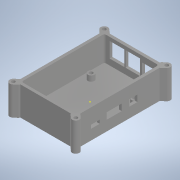
# Autodesk Inventor part: Case Rev D
Saved by Autodesk Inventor 2021 (Build 250183000, 183)
## iProperties
Created: 2021-07-24
Part Number: Case Rev D
Material: ABS Plastic
Document SubType Name: Modeling
Designer: cmzgt
Density: 0.1 g/cm^3
Appearance: Smooth - White
Author: cmzgt
Autodesk Inventor part; units mm, degrees
ref_plane "YZ Plane" through (0, 0, 0) normal (1, 0, 0) x (0, 1, 0)
ref_plane "XZ Plane" through (0, 0, 0) normal (0, 1, 0) x (-1, 0, 0)
ref_plane "XY Plane" through (0, 0, 0) normal (0, 0, 1) x (1, 0, 0)
sketch "Sketch1" plane through (0, 0, 0) normal (0, 1, 0) x (-1, 0, 0)
  line L0 (-33.8, -50.05) -> (33.8, -50.05)
  line L1 (33.8, -50.05) -> (33.8, 50.05)
  line L2 (33.8, 50.05) -> (-33.8, 50.05)
  line L3 (-33.8, 50.05) -> (-33.8, -50.05)
  line L4 (-33.8, -50.05) -> (33.8, 50.05) construction
  line L5 (33.8, -50.05) -> (-33.8, 50.05) construction
  point P0 (0, 0)
  dimension "d0" = 67.6
  dimension "d1" = 100.1
  constraints: 12 end point, 2 midpoint, 2 parallel, 1 horizontal, 1 perpendicular
  measures "d0" distance of L2.end L1.end
  measures "d1" distance of L0.end L1.end
extrude "Extrusion1" add sketch "Sketch1" along normal blind 4.445
sketch "Sketch2" plane through (0, 4.445, 0) normal (0, 1, 0) x (1, 0, 0)
  line L0 (30.6, 46.85) -> (-30.6, 46.85)
  line L1 (-30.6, 46.85) -> (-30.6, -46.85)
  line L2 (-30.6, -46.85) -> (30.6, -46.85)
  line L3 (30.6, -46.85) -> (30.6, 46.85)
  line L4 (30.6, 46.85) -> (-30.6, -46.85) construction
  line L5 (-30.6, 46.85) -> (30.6, -46.85) construction
  line L6 (-33.8, 50.05) -> (-33.8, -50.05) projected
  line L7 (-33.8, -50.05) -> (33.8, -50.05) projected
  line L8 (33.8, 50.05) -> (-33.8, 50.05) projected
  line L9 (33.8, -50.05) -> (33.8, 50.05) projected
  line L10 (27.4, -43.65) -> (33.8, -50.05) construction
  line L11 (24.9431, -46.85) -> (30.9716, -52.8784)
  line L12 (36.6284, -47.2216) -> (30.6, -41.1931)
  arc A0 (30.9716, -52.8784) -> (36.6284, -47.2216) centre (33.8, -50.05) ccw
  circle A1 centre (33.8, -50.05) radius 1.375
  point P0 (0, 0)
  dimension "d4" = 3.2
  dimension "d5" = 3.2
  dimension "d22" = 8
  dimension "d23" = 2.75
  constraints: 20 end point, 4 parallel, 3 midpoint, 2 centre point, 2 point on circle, 2 point on line, 2 tangent, 1 coincident, 1 horizontal, 1 perpendicular
  measures "d4" distance between parallel lines of L6 L1
  measures "d5" distance between parallel lines of L7 L2
  measures "d22" diameter of A0
  measures "d23" diameter of A1
extrude "Extrusion2" add sketch "Sketch2" along normal blind 28 contours L0 L1 L2 L11 L7 L6 L8 L9 L12 L3 | L12 L9 A1 L7 L11 L2 L3 | L9 L7 A1 picked at (32.9402, -49.7491)
sketch "Sketch4" plane through (0, 0, 0) normal (0, -1, 0) x (1, 0, 0)
  line L0 (32.2906, 48.7379) -> (35.3094, 51.3621) construction
  line L1 (33.8, 50.05) -> (33.8, -50.05) projected
  line L2 (33.8, 44.7499) -> (37.9337, 48.3433)
  line L3 (32.6852, 54.381) -> (29.6663, 51.7567)
  arc A0 (29.6663, 51.7567) -> (28.5119, 50.05) centre (32.2906, 48.7379) ccw
  arc A1 (37.9337, 48.3433) -> (32.6852, 54.381) centre (35.3094, 51.3621) ccw
  line L4 (-33.8, 50.05) -> (33.8, 50.05) projected
  line L5 (28.5119, 50.05) -> (33.8, 50.05)
  line L6 (33.8, 50.05) -> (33.8, 44.7499)
  circle A2 centre (35.3094, 51.3621) radius 1.985
  line L7 (0, 50.05) -> (0, -50.05) construction
  line L8 (33.8, -50.05) -> (-33.8, -50.05) construction
  line L9 (33.8, 0) -> (-33.3, 0) construction
  line L10 (33.8, -50.05) -> (33.8, 50.05)
  line L11 (33.8, -44.7499) -> (37.9337, -48.3433)
  line L12 (32.6852, -54.381) -> (29.6663, -51.7567)
  arc A3 (28.5119, -50.05) -> (29.6663, -51.7567) centre (32.2906, -48.7379) ccw
  arc A4 (32.6852, -54.381) -> (37.9337, -48.3433) centre (35.3094, -51.3621) ccw
  line L13 (-33.8, -50.05) -> (33.8, -50.05)
  circle A5 centre (35.3094, -51.3621) radius 1.985
  line L14 (-33.8, 50.05) -> (-33.8, -50.05)
  line L15 (-33.8, 44.7499) -> (-37.9337, 48.3433)
  line L16 (-32.6852, 54.381) -> (-29.6663, 51.7567)
  arc A6 (-28.5119, 50.05) -> (-29.6663, 51.7567) centre (-32.2906, 48.7379) ccw
  arc A7 (-32.6852, 54.381) -> (-37.9337, 48.3433) centre (-35.3094, 51.3621) ccw
  line L17 (-28.5119, 50.05) -> (-33.8, 50.05)
  circle A8 centre (-35.3094, 51.3621) radius 1.985
  arc A9 (-37.9337, -48.3433) -> (-32.6852, -54.381) centre (-35.3094, -51.3621) ccw
  line L18 (-33.8, -44.7499) -> (-37.9337, -48.3433)
  line L19 (-32.6852, -54.381) -> (-29.6663, -51.7567)
  arc A10 (-29.6663, -51.7567) -> (-28.5119, -50.05) centre (-32.2906, -48.7379) ccw
  circle A11 centre (-35.3094, -51.3621) radius 1.985
  line L20 (-28.5119, -50.05) -> (-33.8, -50.05)
  line L21 (-33.8, -50.05) -> (-33.8, 50.05)
  point P0 (0, 0)
  point P1 (-28.5119, -50.05)
  point P2 (-33.8, -44.7499)
  point P3 (-28.5119, 50.05)
  point P4 (33.8, -44.7499)
  dimension "d24" = 2
  dimension "d25" = 8
  dimension "d26" = 131
  dimension "d27" = 3.97
  constraints: 40 end point, 30 symmetric about line, 16 point on circle, 12 centre point, 6 point on line, 4 coincident, 4 midpoint, 4 tangent, 1 collinear, 1 horizontal, 1 parallel, 9 other
  measures "d24" distance of L1.start L0.end
  measures "d25" diameter of A1
  measures "d26" angle of L1 L2
  measures "d27" diameter of A2
extrude "Extrusion4" add sketch "Sketch4" against normal up to surface (32.445 mm away) contours L4 A0 L3 A1 L2 L1 | L11 A4 L12 A3 L13 L1 | L4 L14 L15 A7 L16 A6 | A10 L19 A9 L18 L14 L13
fillet "Fillet2" radius 2 4 edges at (30.6, 18.445, -46.85) (-30.6, 18.445, -46.85) (-30.6, 18.445, 46.85) (30.6, 18.445, 46.85)
sketch "Sketch14" plane through (0, 4.445, 0) normal (0, 1, 0) x (1, 0, 0)
  circle A0 centre (27.1, -34.85) radius 3.7
  circle A1 centre (27.1, -34.85) radius 1.985
  line L0 (28.6, -46.85) -> (-28.6, -46.85) projected
  line L1 (30.6, 44.85) -> (30.6, -44.85) projected
  line L2 (-28.6, -46.85) -> (28.6, -46.85) construction
  line L3 (0, -46.85) -> (0, 50.05) construction
  line L4 (28.5119, 50.05) -> (-28.5119, 50.05) construction
  circle A2 centre (27.1, 23.15) radius 3.7
  circle A3 centre (27.1, 23.15) radius 1.985
  line L5 (-30.6, 44.85) -> (-30.6, -44.85) construction
  line L6 (-30.6, 0) -> (30.6, 0) construction
  line L7 (30.6, -44.85) -> (30.6, 44.85) construction
  circle A4 centre (-21.9, -34.85) radius 3.7
  circle A5 centre (-21.9, -34.85) radius 1.985
  circle A6 centre (-21.9, 23.15) radius 1.985
  circle A7 centre (-21.9, 23.15) radius 3.7
  point P0 (0, 0)
  dimension "d114" = 7.4
  dimension "d115" = 3.97
  dimension "d116" = 12
  dimension "d117" = 3.5
  dimension "d120" = 58
  dimension "d127" = 49
  constraints: 8 centre point, 4 coincident, 4 end point, 4 midpoint, 1 horizontal, 1 vertical, 12 other
  measures "d114" diameter of A0
  measures "d115" diameter of A1
  measures "d116" distance from line of L0 A0.centre
  measures "d117" distance from line of L1 A0.centre
  measures "d120" distance of A0.centre A2.centre
  measures "d127" distance of A0.centre A4.centre
sketch "Sketch15" plane through (0, 4.445, 0) normal (0, 1, 0) x (1, 0, 0)
  point P0 (0, 0)
extrude "Extrusion10" add sketch "Sketch14" along normal blind 6
sketch "Sketch16" plane through (33.8, 0, 44.7499) normal (1, 0, 0) x (0, 0, -1)
  line L0 (12.9515, 13.2621) -> (12.9515, 13.455) projected
  line L1 (20.9323, 13.455) -> (20.9323, 13.2621) projected
  line L2 (13.9419, 14.5004) -> (19.9419, 14.5004) projected
  line L3 (88.3241, 11.975) -> (9.3999, 11.975) projected
  line L4 (21.9323, 11.475) -> (11.9515, 11.475)
  line L5 (11.9515, 11.475) -> (11.9515, 15.5004)
  line L6 (11.9515, 15.5004) -> (21.9323, 15.5004)
  line L7 (21.9323, 15.5004) -> (21.9323, 11.475)
  line L8 (30.8419, 17.055) -> (30.8419, 14.5766) projected
  line L9 (45.8419, 14.5766) -> (45.8419, 17.055) projected
  line L10 (45.0419, 17.855) -> (31.6419, 17.855) projected
  line L11 (46.8419, 11.475) -> (29.8419, 11.475)
  line L12 (29.8419, 11.475) -> (29.8419, 18.855)
  line L13 (29.8419, 18.855) -> (46.8419, 18.855)
  line L14 (46.8419, 18.855) -> (46.8419, 11.475)
  line L15 (56.4419, 17.775) -> (56.4419, 11.775) projected
  line L16 (63.4419, 11.775) -> (63.4419, 17.775) projected
  line L17 (63.4419, 17.775) -> (59.9419, 17.775) projected
  line L18 (59.9419, 17.775) -> (56.4419, 17.775) projected
  line L19 (64.4419, 11.475) -> (55.4419, 11.475)
  line L20 (55.4419, 11.475) -> (55.4419, 18.775)
  line L21 (55.4419, 18.775) -> (64.4419, 18.775)
  line L22 (64.4419, 18.775) -> (64.4419, 11.475)
  point P0 (44.7499, 0)
  dimension "d134" = 1
  dimension "d135" = 0.5
  dimension "d136" = 1
  dimension "d137" = 1
  dimension "d138" = 1
  dimension "d139" = 0.5
  dimension "d140" = 1
  dimension "d141" = 1
  dimension "d142" = 0.5
  dimension "d143" = 1
  dimension "d144" = 1
  dimension "d145" = 1
  constraints: 24 end point, 6 parallel, 3 horizontal, 3 perpendicular
  measures "d134" distance between parallel lines of L2 L6
  measures "d135" distance between parallel lines of L3 L4
  measures "d136" distance between parallel lines of L1 L7
  measures "d137" distance between parallel lines of L5 L0
  measures "d138" distance between parallel lines of L13 L10
  measures "d139" distance between parallel lines of L3 L11
  measures "d140" distance between parallel lines of L9 L14
  measures "d141" distance from line of L8.end L12
  measures "d142" distance between parallel lines of L3 L19
  measures "d143" distance between parallel lines of L16 L22
  measures "d144" distance between parallel lines of L15 L20
  measures "d145" distance between parallel lines of L18 L21
extrude "Extrusion11" cut sketch "Sketch16" against normal up to surface (3.2 mm away)
sketch "Sketch17" plane through (28.5119, 0, -50.05) normal (0, 0, -1) x (-1, 0, 0)
  line L0 (16.1912, 11.975) -> (16.1912, 25.475) projected
  line L1 (0.3112, 11.975) -> (0.3112, 25.475) projected
  line L2 (0.3112, 25.475) -> (16.1912, 25.475) projected
  line L3 (50.9119, 11.975) -> (0.9119, 11.975) projected
  line L4 (16.4912, 11.725) -> (0.0112, 11.725)
  line L5 (0.0112, 11.725) -> (0.0112, 25.725)
  line L6 (0.0112, 25.725) -> (16.4912, 25.725)
  line L7 (16.4912, 25.725) -> (16.4912, 11.725)
  line L8 (19.4512, 18.7546) -> (19.4512, 21.7546) projected
  line L9 (34.5512, 21.7546) -> (34.5512, 18.7546) projected
  line L10 (24.0012, 27.465) -> (30.0012, 27.465) projected
  line L11 (35.2512, 11.225) -> (18.7512, 11.225)
  line L12 (18.7512, 11.225) -> (18.7512, 28.465)
  line L13 (18.7512, 28.465) -> (35.2512, 28.465)
  line L14 (35.2512, 28.465) -> (35.2512, 11.225)
  line L15 (37.4512, 18.7546) -> (37.4512, 21.7546) projected
  line L16 (52.5512, 21.7546) -> (52.5512, 18.7546) projected
  line L17 (42.0012, 27.465) -> (48.0012, 27.465) projected
  line L18 (53.2512, 11.225) -> (36.7512, 11.225)
  line L19 (36.7512, 11.225) -> (36.7512, 28.465)
  line L20 (36.7512, 28.465) -> (53.2512, 28.465)
  line L21 (53.2512, 28.465) -> (53.2512, 11.225)
  point P0 (28.5119, 0)
  point P1 (18.7512, 11.975)
  point P2 (35.2512, 11.975)
  dimension "d148" = 0.3
  dimension "d149" = 0.3
  dimension "d150" = 0.25
  dimension "d151" = 0.25
  dimension "d154" = 0.7
  dimension "d155" = 0.7
  dimension "d156" = 1
  dimension "d157" = 0.75
  dimension "d158" = 1
  dimension "d159" = 0.7
  dimension "d160" = 0.7
  dimension "d161" = 0.75
  constraints: 24 end point, 6 parallel, 3 horizontal, 3 perpendicular
  measures "d148" distance between parallel lines of L1 L5
  measures "d149" distance between parallel lines of L0 L7
  measures "d150" distance between parallel lines of L3 L4
  measures "d151" distance between parallel lines of L2 L6
  measures "d154" distance between parallel lines of L8 L12
  measures "d155" distance between parallel lines of L9 L14
  measures "d156" distance between parallel lines of L10 L13
  measures "d157" distance between parallel lines of L3 L11
  measures "d158" distance between parallel lines of L17 L20
  measures "d159" distance between parallel lines of L15 L19
  measures "d160" distance between parallel lines of L21 L16
  measures "d161" distance between parallel lines of L3 L18
extrude "Extrusion12" cut sketch "Sketch17" against normal up to surface (3.2 mm away)
body "Solid1"
